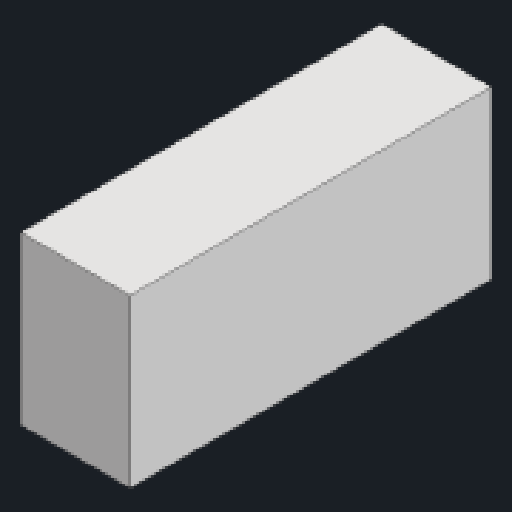
# Autodesk Inventor part: lipo3s650
Saved by Autodesk Inventor 2023 (Build 270158000, 158)
## iProperties
Created: 2024-04-13
Part Number: lipo3s650
Material: Generic
Document SubType Name: Modeling
Designer: szymo
Density: 1 g/cm^3
Appearance: Default
Author: szymo
Autodesk Inventor part; units mm, degrees
ref_plane "YZ Plane" through (0, 0, 0) normal (1, 0, 0) x (0, 1, 0)
ref_plane "XZ Plane" through (0, 0, 0) normal (0, 1, 0) x (-1, 0, 0)
ref_plane "XY Plane" through (0, 0, 0) normal (0, 0, 1) x (1, 0, 0)
sketch "Sketch2" plane through (0, 0, 0) normal (0, 1, 0) x (-1, 0, 0)
  line L0 (0, 0) -> (-20, 0)
  line L1 (-20, 0) -> (-20, -66)
  line L2 (-20, -66) -> (0, -66)
  line L3 (0, -66) -> (0, 0)
  dimension "d0" = 20
  dimension "d1" = 66
  constraints: 8 end point, 2 parallel, 1 horizontal, 1 perpendicular
  measures "d0" distance of L2.end L1.end
  measures "d1" distance of L1.end L0.end
extrude "Extrusion1" add sketch "Sketch2" along normal blind 30.5
sketch "Sketch3" plane through (20, 0, 0) normal (1, 0, 0) x (0, 0, -1)
  line L0 (39.4, 20.369) -> (34.4, 20.369) projected
  line L1 (39.4, 10.125) -> (34.4, 10.125) projected
  line L2 (34.4, 18.9168) -> (34.4, 10.625) projected
  line L3 (34.4, 20.369) -> (34.4, 18.9308) projected
  line L4 (0, 0) -> (0, 30.5) projected
  line L5 (34.4, 20.369) -> (0, 20.369)
  line L6 (0, 20.369) -> (0, 10.125)
  line L7 (0, 10.125) -> (34.4, 10.125)
  line L8 (34.4, 10.125) -> (34.4, 20.369)
  constraints: 8 end point, 2 parallel, 1 horizontal, 1 perpendicular, 1 point on line
ref_plane "Work Plane1" through (25.25, 10.625, -39.4) normal (1, 0, 0) x (0, 1, 0)
extrude "Extrusion2" add sketch "Sketch3" along normal up to surface (5.25 mm away)
body "Solid1"
